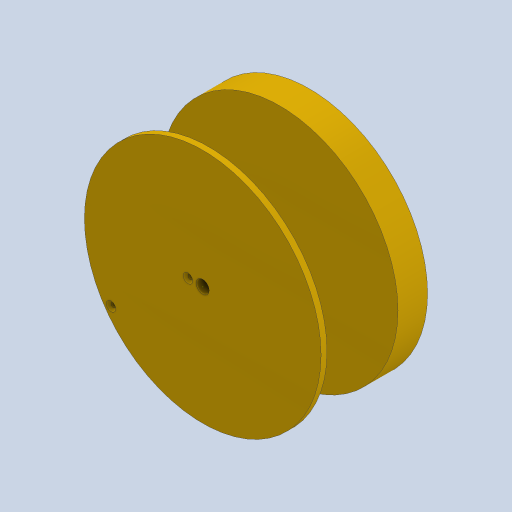
# Autodesk Inventor part: Bobbin_z
Saved by Autodesk Inventor 2024 (Build 280153000, 153)
## iProperties
Created: 2022-01-24
Part Number: Bobbin_z
Material: Generic
Document SubType Name: Modeling
Designer: frede
Density: 1 g/cm^3
Appearance: Default
Author: frede
Autodesk Inventor part; units mm, degrees
ref_plane "YZ Plane" through (0, 0, 0) normal (1, 0, 0) x (0, 1, 0)
ref_plane "XZ Plane" through (0, 0, 0) normal (0, 1, 0) x (-1, 0, 0)
ref_plane "XY Plane" through (0, 0, 0) normal (0, 0, 1) x (1, 0, 0)
sketch "Sketch1" plane through (0, 0, 0) normal (0, 0, 1) x (1, 0, 0)
  circle A0 centre (0, 0) radius 20
  dimension "d0" = 40
  constraints: 1 centre point, 1 coincident
  measures "d0" diameter of A0
extrude "Extrusion1" add sketch "Sketch1" along normal blind 5
sketch "Sketch2" plane through (0, 0, 5) normal (0, 0, 1) x (1, 0, 0)
  circle A0 centre (0, 0) radius 2
  dimension "d3" = 4
  constraints: 1 centre point, 1 coincident
  measures "d3" diameter of A0
extrude "Extrusion2" add sketch "Sketch2" along normal blind 12
sketch "Sketch3" plane through (0, 0, 17) normal (0, 0, 1) x (1, 0, 0)
  circle A0 centre (0, 0) radius 20
  dimension "d6" = 40
  constraints: 1 centre point, 1 coincident
  measures "d6" diameter of A0
extrude "Extrusion3" add sketch "Sketch3" along normal blind 1
sketch "Sketch4" plane through (0, 0, 18) normal (0, 0, 1) x (1, 0, 0)
  circle A0 centre (0, 0) radius 1.1
  dimension "d9" = 2.2
  constraints: 1 centre point, 1 coincident
  measures "d9" diameter of A0
extrude "Extrusion4" cut sketch "Sketch4" against normal through all
sketch "Sketch6" plane through (0, 0, 18) normal (0, 0, 1) x (1, 0, 0)
  circle A0 centre (0, 0) radius 2 construction
  circle A1 centre (-15.5, -10.6066) radius 0.4
  circle A2 centre (-2.5, 0) radius 0.4
  circle A3 centre (0, 0) radius 20 projected
  dimension "d20" = 0.8
  dimension "d21" = 0.8
  dimension "d38" = 2.5
  dimension "d39" = 15.5
  constraints: 2 centre point
  measures "d20" diameter of A1
  measures "d21" diameter of A2
  measures "d38" distance of A0.centre A2.centre
  measures "d39" horizontal distance of A3.centre A1.centre
sketch "Sketch7" plane through (0, 0, 18) normal (0, 0, 1) x (1, 0, 0)
  point P0 (0, 0)
extrude "Extrusion5" cut sketch "Sketch6" against normal up to surface (1 mm away) contours A1 | A2
chamfer "Chamfer1" distance 0.4 angle 45 2 edges at (-2.9, 0, 18) (-15.9, -10.6066, 18)
sketch "Sketch11" plane through (0, 0, 0) normal (0, 0, -1) x (-1, 0, 0)
  circle A0 centre (0, 0) radius 20 projected
  point P0 (-5, 26.5)
  point P1 (-5, -26.5)
  dimension "d40" = 26.5
  dimension "d41" = 5
  dimension "d42" = 5
  dimension "d43" = 26.5
  measures "d40" vertical distance of A0.centre point (-5, -26.5)
  measures "d41" horizontal distance of point (0, 0) point (-5, -26.5)
  measures "d42" horizontal distance of point (0, 0) point (-5, 26.5)
  measures "d43" vertical distance of point (0, 0) point (-5, 26.5)
hole "Hole3" at (5, -26.5, 0) at (5, 26.5, 0) direction (0, 0, 1) diameter 1.567 end through all thread size "M2x0.4" class "6H" standard "ISO Metric profile"
sketch "Sketch12" plane through (0, 0, 0) normal (0, 0, -1) x (-1, 0, 0)
  point P0 (0, 0)
  point P1 (5, 0)
  point P2 (-5, 0)
  dimension "d55" = 5
  dimension "d56" = 5
  measures "d55" distance of point (0, 0) point (5, 0)
  measures "d56" distance of point (0, 0) point (-5, 0)
hole "Hole4" at (-5, 0, 0) at (5, 0, 0) direction (0, 0, 1) diameter 2.459 depth 4.8 thread size "M3x0.5" class "6H" standard "ISO Metric profile"
loft "Loft1" [suppressed]
body "Solid1"
body "Solid2"
